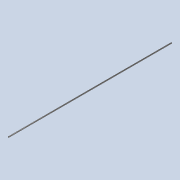
# Autodesk Inventor part: String
Saved by Autodesk Inventor 2021 (Build 250183000, 183)
## iProperties
Created: 2021-03-17
Part Number: String
Material: Stainless Steel
Document SubType Name: Modeling
Designer: Tom
Density: 8 g/cm^3
Appearance: Semi-Polished
Author: Tom
Autodesk Inventor part; units mm, degrees
ref_plane "YZ Plane" through (0, 0, 0) normal (1, 0, 0) x (0, 1, 0)
ref_plane "XZ Plane" through (0, 0, 0) normal (0, 1, 0) x (-1, 0, 0)
ref_plane "XY Plane" through (0, 0, 0) normal (0, 0, 1) x (1, 0, 0)
sketch "Sketch1" plane through (0, 0, 0) normal (0, 0, 1) x (1, 0, 0)
  circle A0 centre (0, 0) radius 0.7937
  line L0 (-0.7937, 0.7937) -> (0.7937, 0.7938)
  line L1 (0.7937, 0.7938) -> (0.7937, -0.7937)
  line L2 (0.7937, -0.7937) -> (-0.7937, -0.7937)
  line L3 (-0.7937, -0.7937) -> (-0.7937, 0.7937)
  point P0 (-0.7937, 0)
  point P1 (0, -0.7937)
  point P2 (0, 0.7937)
  point P3 (0.7937, 0)
  dimension "d0" = 1.5875
  constraints: 8 end point, 4 tangent, 2 parallel, 1 centre point, 1 coincident, 1 horizontal, 1 perpendicular
  measures "d0" diameter of A0
extrude "Extrusion1" add sketch "Sketch1" against normal blind 463.55
body "Solid1"
